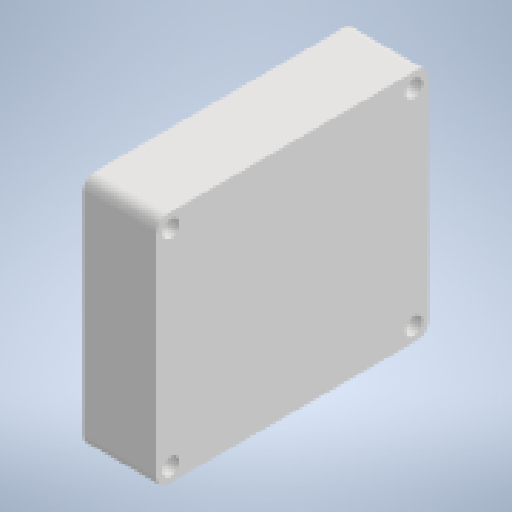
# Autodesk Inventor part: MDD3A
Saved by Autodesk Inventor 2025.2 (Build 292293000, 293)
## iProperties
Created: 2025-02-22
Part Number: MDD3A
Material: Générique
Document SubType Name: Modeling
Designer: antoi
Density: 1 g/cm^3
Appearance: Par défaut
Author: antoi
Autodesk Inventor part; units mm, degrees
ref_plane "YZ Plane" through (0, 0, 0) normal (1, 0, 0) x (0, 1, 0)
ref_plane "XZ Plane" through (0, 0, 0) normal (0, 1, 0) x (-1, 0, 0)
ref_plane "XY Plane" through (0, 0, 0) normal (0, 0, 1) x (1, 0, 0)
sketch "Esquisse1" plane through (0, 0, 0) normal (1, 0, 0) x (0, 1, 0)
  line L0 (2, 0) -> (39.66, 0)
  line L1 (41.66, -2) -> (41.66, -46.26)
  line L2 (39.66, -48.26) -> (2, -48.26)
  line L3 (0, -46.26) -> (0, -2)
  arc A0 (41.66, -2) -> (39.66, 0) centre (39.66, -2) ccw
  arc A1 (39.66, -48.26) -> (41.66, -46.26) centre (39.66, -46.26) ccw
  arc A2 (0, -46.26) -> (2, -48.26) centre (2, -46.26) ccw
  arc A3 (2, 0) -> (0, -2) centre (2, -2) ccw
  circle A4 centre (2.54, -2.54) radius 1.5
  circle A5 centre (2.54, -45.72) radius 1.5
  circle A6 centre (39.12, -2.54) radius 1.5
  circle A7 centre (39.12, -45.72) radius 1.5
  point P0 (0, 0)
  point P1 (41.66, -48.26)
  point P2 (41.66, 0)
  point P3 (0, -48.26)
  dimension "d0" = 41.66
  dimension "d1" = 48.26
  dimension "d2" = 2
  dimension "d3" = 3
  dimension "d6" = 43.18
  dimension "d9" = 36.58
  constraints: 8 centre point, 8 end point, 8 point on circle, 8 point on line, 8 tangent, 3 equal radius, 2 horizontal, 2 parallel, 1 perpendicular, 1 vertical, 6 other
  measures "d0" distance of point (41.66, -48.26) point (0, -48.26)
  measures "d1" distance of point (41.66, 0) point (41.66, -48.26)
  measures "d2" radius of A0
  measures "d3" diameter of A4
  measures "d6" distance of A4.centre A5.centre
  measures "d9" distance of A4.centre A6.centre
extrude "Extrusion1" add sketch "Esquisse1" along normal blind 13
